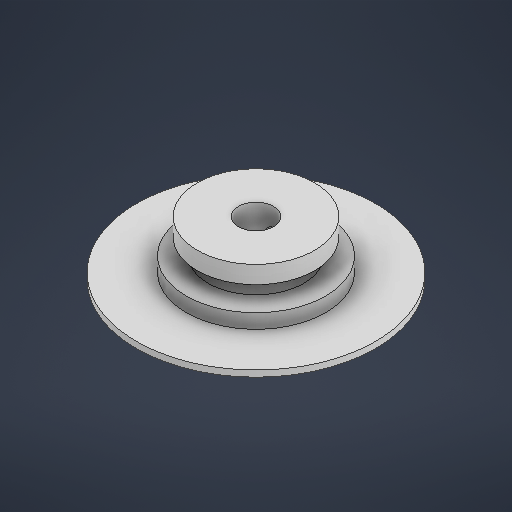
# Autodesk Inventor part: encoder wheel
Saved by Autodesk Inventor 2025.2 (Build 292293000, 293)
## iProperties
Created: 2025-04-19
Part Number: encoder wheel
Material: Generic
Document SubType Name: Modeling
Designer: klawy
Density: 1 g/cm^3
Appearance: Default
Author: klawy
Autodesk Inventor part; units mm, degrees
ref_plane "YZ Plane" through (0, 0, 0) normal (1, 0, 0) x (0, 1, 0)
ref_plane "XZ Plane" through (0, 0, 0) normal (0, 1, 0) x (-1, 0, 0)
ref_plane "XY Plane" through (0, 0, 0) normal (0, 0, 1) x (1, 0, 0)
sketch "Sketch2" plane through (0, 0, 0) normal (0, 0, 1) x (1, 0, 0)
  line L0 (-13.335, 16.8924) -> (13.335, 16.8924) construction
  line L1 (13.335, 16.8924) -> (13.335, 20.8924)
  line L2 (13.335, 20.8924) -> (-13.335, 20.8924) construction
  line L3 (-13.335, 20.8924) -> (-13.335, 16.8924)
  line L4 (-13.335, 16.8924) -> (13.335, 20.8924) construction
  line L5 (13.335, 16.8924) -> (-13.335, 20.8924) construction
  line L6 (0, -12.1762) -> (0, 12.1762) construction
  line L7 (-9, 16.8924) -> (9, 16.8924) construction
  line L8 (9, 16.8924) -> (9, 20.8924)
  line L9 (9, 20.8924) -> (-9, 20.8924) construction
  line L10 (-9, 20.8924) -> (-9, 16.8924)
  line L11 (-9, 16.8924) -> (9, 20.8924) construction
  line L12 (9, 16.8924) -> (-9, 20.8924) construction
  line L13 (31.2915, 53.5117) -> (31.2915, -42.8656) construction
  line L14 (31.2915, -42.8656) -> (-90.5187, -42.8656) construction
  line L15 (-90.5187, -42.8656) -> (-90.5187, 53.5117) construction
  line L16 (-90.5187, 53.5117) -> (31.2915, 53.5117) construction
  line L17 (15.8601, 8.4424) -> (-15.8601, 8.4424)
  line L18 (-15.8601, 8.4424) -> (-15.8601, 13.1433)
  line L19 (-15.8601, 13.1433) -> (15.8601, 13.1433)
  line L20 (15.8601, 13.1433) -> (15.8601, 8.4424)
  line L21 (15.8601, 8.4424) -> (-15.8601, 13.1433) construction
  line L22 (-15.8601, 8.4424) -> (15.8601, 13.1433) construction
  line L23 (27.2146, 8.4512) -> (-27.2146, 8.4512)
  line L24 (-27.2146, 8.4512) -> (-27.2146, 9.8628)
  line L25 (-27.2146, 9.8628) -> (27.2146, 9.8628)
  line L26 (27.2146, 9.8628) -> (27.2146, 8.4512)
  line L27 (27.2146, 8.4512) -> (-27.2146, 9.8628) construction
  line L28 (-27.2146, 8.4512) -> (27.2146, 9.8628) construction
  line L29 (12.0218, 5.3333) -> (-12.0218, 5.3333)
  line L30 (-12.0218, 5.3333) -> (-12.0218, 8.8452)
  line L31 (-12.0218, 8.8452) -> (12.0218, 8.8452)
  line L32 (12.0218, 8.8452) -> (12.0218, 5.3333)
  line L33 (12.0218, 5.3333) -> (-12.0218, 8.8452) construction
  line L34 (-12.0218, 5.3333) -> (12.0218, 8.8452) construction
  line L35 (-9, 16.8924) -> (-9, 13.1433)
  line L36 (-9, 15.0178) -> (-10.8745, 13.1433)
  line L37 (9, 16.8924) -> (9, 13.1433)
  line L38 (9, 15.0178) -> (10.8745, 13.1433)
  line L39 (-13.335, 20.8924) -> (13.335, 20.8924)
  line L40 (4, 3.8577) -> (-4, 3.8577) construction
  line L41 (-4, 3.8577) -> (-4, 22.4289)
  line L42 (-4, 22.4289) -> (4, 22.4289) construction
  line L43 (4, 22.4289) -> (4, 3.8577)
  line L44 (4, 3.8577) -> (-4, 22.4289) construction
  line L45 (-4, 3.8577) -> (4, 22.4289) construction
  line L46 (-13.335, 16.8924) -> (13.335, 16.8924)
  point P0 (0, 0)
  point P1 (0, 18.8924)
  point P2 (0, 0)
  point P3 (0, 10.7928)
  point P4 (0, 9.157)
  point P5 (0, 7.0892)
  point P6 (0, 13.1433)
  point P7 (4, 8.4424)
  point P8 (4, 5.3333)
  point P9 (12.0218, 8.4424)
  point P10 (4, 20.8924)
  point P11 (4, 8.4512)
  point P12 (15.8601, 9.8628)
  dimension "d0" = 26.67
  dimension "d1" = 18
  dimension "d32" = 45
  dimension "d33" = 45
  dimension "d36" = 8
  dimension "d44" = 4
  constraints: 86 end point, 16 midpoint, 12 parallel, 10 point on line, 8 perpendicular, 6 horizontal, 2 collinear, 2 vertical, 1 coincident, 2 other
  measures "d0" distance between parallel lines of L1 L3
  measures "d1" distance between parallel lines of L10 L8
  measures "d32" angle of L36 L35
  measures "d33" angle of L37 L38
  measures "d36" distance of L41.end L42.end
  measures "d44" distance of L0.end L1.end
revolve "Revolution1" add sketch "Sketch2" angle 360 about axis through (0, -12.1762, 0) along (0, 1, 0) contours L46 L8 L39 L1 | L46 L43 L39 L8 | L37 L19 L43 L46 | L38 L19 L37 | L19 L20 L25 L43 | L25 L20 L23 L32 L31 L43 | L25 L26 L23 L20 | L31 L32 L23 L43 | L17 L32 L29 L43
sketch "Sketch3" plane through (0, 0, 0) normal (0, 0, 1) x (1, 0, 0)
  line L0 (9, 15.0178) -> (-9, 15.0178) projected
  point P0 (0, 0)
  point P1 (0, 15.0178)
  constraints: 1 midpoint
hole "Hole1" at (0, 15.0178, 0) direction (0, 0, -1) diameter 3.4 end through all clearance for "Hex Head Cap Screw ISO 24017" size "M3" standard "ISO"
body "Solid1"
